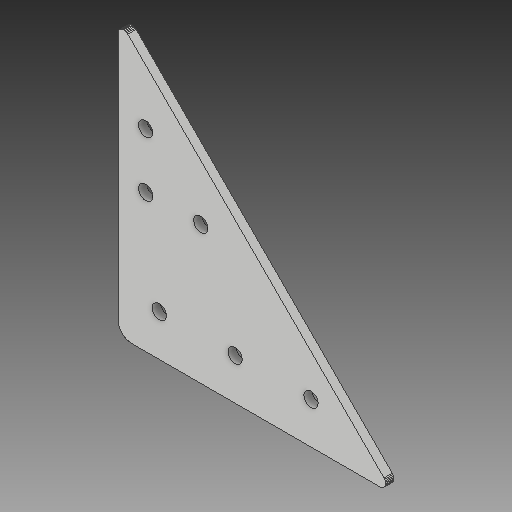
# Autodesk Inventor part: Side Brace
Saved by Autodesk Inventor 2018 (Build 220112000, 112)
## iProperties
Created: 2016-07-21
Part Number: Side Brace
Material: Generic
Document SubType Name: Modeling
Designer: User
Density: 1 g/cm^3
Appearance: Default
Author: User
Autodesk Inventor part; units mm, degrees
ref_plane "YZ Plane" through (0, 0, 0) normal (1, 0, 0) x (0, 1, 0)
ref_plane "XZ Plane" through (0, 0, 0) normal (0, 1, 0) x (-1, 0, 0)
ref_plane "XY Plane" through (0, 0, 0) normal (0, 0, 1) x (1, 0, 0)
sketch "Sketch1" plane through (0, 0, 0) normal (0, 0, 1) x (1, 0, 0)
  line L0 (141.1705, 404.7157) -> (141.0527, 405.1042)
  line L1 (141.0527, 405.1042) -> (140.8612, 405.4623)
  line L2 (140.8612, 405.4623) -> (140.6037, 405.7761)
  line L3 (140.6037, 405.7761) -> (47.6678, 498.6981)
  line L4 (47.6678, 498.6981) -> (47.354, 498.9557)
  line L5 (47.354, 498.9557) -> (46.9959, 499.1471)
  line L6 (46.9959, 499.1471) -> (46.6074, 499.265)
  line L7 (46.6074, 499.265) -> (46.2034, 499.3048)
  line L8 (46.2034, 499.3048) -> (45.7993, 499.265)
  line L9 (45.7993, 499.265) -> (45.4108, 499.1471)
  line L10 (45.4108, 499.1471) -> (45.0528, 498.9557)
  line L11 (45.0528, 498.9557) -> (44.7389, 498.6982)
  line L12 (44.7389, 498.6982) -> (44.4814, 498.3843)
  line L13 (44.4814, 498.3843) -> (44.29, 498.0263)
  line L14 (44.29, 498.0263) -> (44.1721, 497.6378)
  line L15 (44.1721, 497.6378) -> (44.1323, 497.2337)
  line L16 (44.1323, 497.2337) -> (44.1323, 407.2337)
  line L17 (44.1323, 407.2337) -> (44.1751, 406.5811)
  line L18 (44.1751, 406.5811) -> (44.3027, 405.9396)
  line L19 (44.3027, 405.9396) -> (44.5129, 405.3203)
  line L20 (44.5129, 405.3203) -> (44.8022, 404.7337)
  line L21 (44.8022, 404.7337) -> (45.1655, 404.1899)
  line L22 (45.1655, 404.1899) -> (45.5968, 403.6982)
  line L23 (45.5968, 403.6982) -> (46.0885, 403.2669)
  line L24 (46.0885, 403.2669) -> (46.6323, 402.9036)
  line L25 (46.6323, 402.9036) -> (47.2189, 402.6143)
  line L26 (47.2189, 402.6143) -> (47.8382, 402.4041)
  line L27 (47.8382, 402.4041) -> (48.4797, 402.2765)
  line L28 (48.4797, 402.2765) -> (49.1323, 402.2337)
  line L29 (49.1323, 402.2337) -> (139.1323, 402.2337)
  line L30 (139.1323, 402.2337) -> (139.5404, 402.2701)
  line L31 (139.5404, 402.2701) -> (139.929, 402.3879)
  line L32 (139.929, 402.3879) -> (140.287, 402.5794)
  line L33 (140.287, 402.5794) -> (140.6008, 402.8369)
  line L34 (140.6008, 402.8369) -> (140.8618, 403.1549)
  line L35 (140.8618, 403.1549) -> (141.0532, 403.513)
  line L36 (141.0532, 403.513) -> (141.1711, 403.9015)
  line L37 (141.1711, 403.9015) -> (141.2109, 404.3055)
  line L38 (141.2109, 404.3055) -> (141.1705, 404.7157)
  line L39 (89.0593, 417.8849) -> (88.8076, 418.4926)
  line L40 (88.8076, 418.4926) -> (88.4071, 419.0145)
  line L41 (88.4071, 419.0145) -> (87.8852, 419.415)
  line L42 (87.8852, 419.415) -> (87.2774, 419.6668)
  line L43 (87.2774, 419.6668) -> (86.6252, 419.7526)
  line L44 (86.6252, 419.7526) -> (85.973, 419.6669)
  line L45 (85.973, 419.6669) -> (85.3652, 419.4151)
  line L46 (85.3652, 419.4151) -> (84.8433, 419.0147)
  line L47 (84.8433, 419.0147) -> (84.4428, 418.4928)
  line L48 (84.4428, 418.4928) -> (84.1911, 417.885)
  line L49 (84.1911, 417.885) -> (84.1052, 417.2328)
  line L50 (84.1052, 417.2328) -> (84.191, 416.5805)
  line L51 (84.191, 416.5805) -> (84.4427, 415.9728)
  line L52 (84.4427, 415.9728) -> (84.8432, 415.4509)
  line L53 (84.8432, 415.4509) -> (85.3651, 415.0503)
  line L54 (85.3651, 415.0503) -> (85.9728, 414.7986)
  line L55 (85.9728, 414.7986) -> (86.6251, 414.7128)
  line L56 (86.6251, 414.7128) -> (87.2773, 414.7985)
  line L57 (87.2773, 414.7985) -> (87.8851, 415.0503)
  line L58 (87.8851, 415.0503) -> (88.407, 415.4507)
  line L59 (88.407, 415.4507) -> (88.8075, 415.9726)
  line L60 (88.8075, 415.9726) -> (89.0592, 416.5803)
  line L61 (89.0592, 416.5803) -> (89.1451, 417.2326)
  line L62 (89.1451, 417.2326) -> (89.0593, 417.8849)
  line L63 (61.5613, 417.885) -> (61.3095, 418.4929)
  line L64 (61.3095, 418.4929) -> (60.9091, 419.0148)
  line L65 (60.9091, 419.0148) -> (60.3872, 419.4153)
  line L66 (60.3872, 419.4153) -> (59.7794, 419.667)
  line L67 (59.7794, 419.667) -> (59.1271, 419.7529)
  line L68 (59.1271, 419.7529) -> (58.4749, 419.6671)
  line L69 (58.4749, 419.6671) -> (57.8671, 419.4154)
  line L70 (57.8671, 419.4154) -> (57.3452, 419.0149)
  line L71 (57.3452, 419.0149) -> (56.9447, 418.493)
  line L72 (56.9447, 418.493) -> (56.693, 417.8853)
  line L73 (56.693, 417.8853) -> (56.6071, 417.233)
  line L74 (56.6071, 417.233) -> (56.6929, 416.5808)
  line L75 (56.6929, 416.5808) -> (56.9446, 415.973)
  line L76 (56.9446, 415.973) -> (57.3451, 415.4511)
  line L77 (57.3451, 415.4511) -> (57.867, 415.0506)
  line L78 (57.867, 415.0506) -> (58.4748, 414.7989)
  line L79 (58.4748, 414.7989) -> (59.127, 414.713)
  line L80 (59.127, 414.713) -> (59.7792, 414.7988)
  line L81 (59.7792, 414.7988) -> (60.387, 415.0505)
  line L82 (60.387, 415.0505) -> (60.9089, 415.451)
  line L83 (60.9089, 415.451) -> (61.3094, 415.9729)
  line L84 (61.3094, 415.9729) -> (61.5611, 416.5806)
  line L85 (61.5611, 416.5806) -> (61.647, 417.233)
  line L86 (61.647, 417.233) -> (61.5613, 417.885)
  line L87 (56.5942, 452.8937) -> (56.3395, 453.5086)
  line L88 (56.3395, 453.5086) -> (55.9343, 454.0367)
  line L89 (55.9343, 454.0367) -> (55.4062, 454.4419)
  line L90 (55.4062, 454.4419) -> (54.7911, 454.6967)
  line L91 (54.7911, 454.6967) -> (54.1311, 454.7836)
  line L92 (54.1311, 454.7836) -> (53.4711, 454.6968)
  line L93 (53.4711, 454.6968) -> (52.8561, 454.4421)
  line L94 (52.8561, 454.4421) -> (52.328, 454.0368)
  line L95 (52.328, 454.0368) -> (51.9227, 453.5087)
  line L96 (51.9227, 453.5087) -> (51.668, 452.8937)
  line L97 (51.668, 452.8937) -> (51.5811, 452.2338)
  line L98 (51.5811, 452.2338) -> (51.6679, 451.5738)
  line L99 (51.6679, 451.5738) -> (51.9226, 450.9587)
  line L100 (51.9226, 450.9587) -> (52.3279, 450.4306)
  line L101 (52.3279, 450.4306) -> (52.856, 450.0253)
  line L102 (52.856, 450.0253) -> (53.471, 449.7706)
  line L103 (53.471, 449.7706) -> (54.131, 449.6837)
  line L104 (54.131, 449.6837) -> (54.791, 449.7705)
  line L105 (54.791, 449.7705) -> (55.406, 450.0252)
  line L106 (55.406, 450.0252) -> (55.9341, 450.4305)
  line L107 (55.9341, 450.4305) -> (56.3394, 450.9586)
  line L108 (56.3394, 450.9586) -> (56.5941, 451.5736)
  line L109 (56.5941, 451.5736) -> (56.681, 452.2337)
  line L110 (56.681, 452.2337) -> (56.5942, 452.8937)
  line L111 (56.597, 472.894) -> (56.3423, 473.509)
  line L112 (56.3423, 473.509) -> (55.9371, 474.0371)
  line L113 (55.9371, 474.0371) -> (55.409, 474.4424)
  line L114 (55.409, 474.4424) -> (54.794, 474.6971)
  line L115 (54.794, 474.6971) -> (54.1339, 474.784)
  line L116 (54.1339, 474.784) -> (53.4739, 474.6972)
  line L117 (53.4739, 474.6972) -> (52.8589, 474.4425)
  line L118 (52.8589, 474.4425) -> (52.3308, 474.0372)
  line L119 (52.3308, 474.0372) -> (51.9255, 473.5091)
  line L120 (51.9255, 473.5091) -> (51.6708, 472.8941)
  line L121 (51.6708, 472.8941) -> (51.5839, 472.2341)
  line L122 (51.5839, 472.2341) -> (51.6707, 471.5741)
  line L123 (51.6707, 471.5741) -> (51.9254, 470.9591)
  line L124 (51.9254, 470.9591) -> (52.3307, 470.431)
  line L125 (52.3307, 470.431) -> (52.8588, 470.0257)
  line L126 (52.8588, 470.0257) -> (53.4738, 469.771)
  line L127 (53.4738, 469.771) -> (54.1337, 469.6841)
  line L128 (54.1337, 469.6841) -> (54.7938, 469.7709)
  line L129 (54.7938, 469.7709) -> (55.4087, 470.0256)
  line L130 (55.4087, 470.0256) -> (55.9369, 470.4309)
  line L131 (55.9369, 470.4309) -> (56.3422, 470.959)
  line L132 (56.3422, 470.959) -> (56.5969, 471.574)
  line L133 (56.5969, 471.574) -> (56.6838, 472.2341)
  line L134 (56.6838, 472.2341) -> (56.597, 472.894)
  line L135 (76.5952, 452.8937) -> (76.3405, 453.5086)
  line L136 (76.3405, 453.5086) -> (75.9352, 454.0368)
  line L137 (75.9352, 454.0368) -> (75.4071, 454.442)
  line L138 (75.4071, 454.442) -> (74.7921, 454.6968)
  line L139 (74.7921, 454.6968) -> (74.1322, 454.7837)
  line L140 (74.1322, 454.7837) -> (73.4722, 454.6969)
  line L141 (73.4722, 454.6969) -> (72.8571, 454.4421)
  line L142 (72.8571, 454.4421) -> (72.329, 454.0369)
  line L143 (72.329, 454.0369) -> (71.9237, 453.5088)
  line L144 (71.9237, 453.5088) -> (71.669, 452.8938)
  line L145 (71.669, 452.8938) -> (71.5821, 452.2338)
  line L146 (71.5821, 452.2338) -> (71.6689, 451.5738)
  line L147 (71.6689, 451.5738) -> (71.9237, 450.9588)
  line L148 (71.9237, 450.9588) -> (72.3289, 450.4307)
  line L149 (72.3289, 450.4307) -> (72.857, 450.0254)
  line L150 (72.857, 450.0254) -> (73.472, 449.7706)
  line L151 (73.472, 449.7706) -> (74.132, 449.6838)
  line L152 (74.132, 449.6838) -> (74.792, 449.7705)
  line L153 (74.792, 449.7705) -> (75.407, 450.0253)
  line L154 (75.407, 450.0253) -> (75.9352, 450.4305)
  line L155 (75.9352, 450.4305) -> (76.3404, 450.9586)
  line L156 (76.3404, 450.9586) -> (76.5952, 451.5736)
  line L157 (76.5952, 451.5736) -> (76.682, 452.2334)
  line L158 (76.682, 452.2334) -> (76.5952, 452.8937)
  line L159 (116.5587, 417.8849) -> (116.307, 418.4926)
  line L160 (116.307, 418.4926) -> (115.9066, 419.0145)
  line L161 (115.9066, 419.0145) -> (115.3847, 419.415)
  line L162 (115.3847, 419.415) -> (114.7769, 419.6667)
  line L163 (114.7769, 419.6667) -> (114.1247, 419.7526)
  line L164 (114.1247, 419.7526) -> (113.4724, 419.6668)
  line L165 (113.4724, 419.6668) -> (112.8647, 419.415)
  line L166 (112.8647, 419.415) -> (112.3428, 419.0146)
  line L167 (112.3428, 419.0146) -> (111.9423, 418.4927)
  line L168 (111.9423, 418.4927) -> (111.6905, 417.8849)
  line L169 (111.6905, 417.8849) -> (111.6047, 417.2327)
  line L170 (111.6047, 417.2327) -> (111.6904, 416.5804)
  line L171 (111.6904, 416.5804) -> (111.9422, 415.9727)
  line L172 (111.9422, 415.9727) -> (112.3426, 415.4508)
  line L173 (112.3426, 415.4508) -> (112.8645, 415.0503)
  line L174 (112.8645, 415.0503) -> (113.4723, 414.7986)
  line L175 (113.4723, 414.7986) -> (114.1246, 414.7127)
  line L176 (114.1246, 414.7127) -> (114.7768, 414.7985)
  line L177 (114.7768, 414.7985) -> (115.3846, 415.0502)
  line L178 (115.3846, 415.0502) -> (115.9065, 415.4507)
  line L179 (115.9065, 415.4507) -> (116.307, 415.9726)
  line L180 (116.307, 415.9726) -> (116.5587, 416.5802)
  line L181 (116.5587, 416.5802) -> (116.6445, 417.2325)
  line L182 (116.6445, 417.2325) -> (116.5587, 417.8849)
  point P0 (0, 0)
  constraints: 366 end point, 13 perpendicular, 2 parallel
extrude "Extrusion1" add sketch "Sketch1" along normal blind 3
sketch "Sketch2" plane through (0, 0, 0) normal (0, 0, -1) x (-1, 0, 0)
  line L0 (-56.6838, 472.2341) -> (-56.597, 472.894) projected
  line L1 (-56.597, 472.894) -> (-56.3423, 473.509) projected
  line L2 (-56.3423, 473.509) -> (-55.9371, 474.0371) projected
  line L3 (-55.9371, 474.0371) -> (-55.409, 474.4424) projected
  line L4 (-55.409, 474.4424) -> (-54.794, 474.6971) projected
  line L5 (-54.794, 474.6971) -> (-54.1339, 474.784) projected
  line L6 (-54.1339, 474.784) -> (-53.4739, 474.6972) projected
  line L7 (-53.4739, 474.6972) -> (-52.8589, 474.4425) projected
  line L8 (-52.8589, 474.4425) -> (-52.3308, 474.0372) projected
  line L9 (-52.3308, 474.0372) -> (-51.9255, 473.5091) projected
  line L10 (-51.9255, 473.5091) -> (-51.6708, 472.8941) projected
  line L11 (-51.6708, 472.8941) -> (-51.5839, 472.2341) projected
  line L12 (-51.5839, 472.2341) -> (-51.6707, 471.5741) projected
  line L13 (-51.6707, 471.5741) -> (-51.9254, 470.9591) projected
  line L14 (-51.9254, 470.9591) -> (-52.3307, 470.431) projected
  line L15 (-52.3307, 470.431) -> (-52.8588, 470.0257) projected
  line L16 (-52.8588, 470.0257) -> (-53.4738, 469.771) projected
  line L17 (-53.4738, 469.771) -> (-54.1337, 469.6841) projected
  line L18 (-54.1337, 469.6841) -> (-54.7938, 469.7709) projected
  line L19 (-54.7938, 469.7709) -> (-55.4087, 470.0256) projected
  line L20 (-55.4087, 470.0256) -> (-55.9369, 470.4309) projected
  line L21 (-55.9369, 470.4309) -> (-56.3422, 470.959) projected
  line L22 (-56.3422, 470.959) -> (-56.5969, 471.574) projected
  line L23 (-56.5969, 471.574) -> (-56.6838, 472.2341) projected
  line L24 (-76.682, 452.2334) -> (-76.5952, 452.8937) projected
  line L25 (-76.5952, 452.8937) -> (-76.3405, 453.5086) projected
  line L26 (-76.3405, 453.5086) -> (-75.9352, 454.0368) projected
  line L27 (-75.9352, 454.0368) -> (-75.4071, 454.442) projected
  line L28 (-75.4071, 454.442) -> (-74.7921, 454.6968) projected
  line L29 (-74.7921, 454.6968) -> (-74.1322, 454.7837) projected
  line L30 (-74.1322, 454.7837) -> (-73.4722, 454.6969) projected
  line L31 (-73.4722, 454.6969) -> (-72.8571, 454.4421) projected
  line L32 (-72.8571, 454.4421) -> (-72.329, 454.0369) projected
  line L33 (-72.329, 454.0369) -> (-71.9237, 453.5088) projected
  line L34 (-71.9237, 453.5088) -> (-71.669, 452.8938) projected
  line L35 (-71.669, 452.8938) -> (-71.5821, 452.2338) projected
  line L36 (-71.5821, 452.2338) -> (-71.6689, 451.5738) projected
  line L37 (-71.6689, 451.5738) -> (-71.9237, 450.9588) projected
  line L38 (-71.9237, 450.9588) -> (-72.3289, 450.4307) projected
  line L39 (-72.3289, 450.4307) -> (-72.857, 450.0254) projected
  line L40 (-72.857, 450.0254) -> (-73.472, 449.7706) projected
  line L41 (-73.472, 449.7706) -> (-74.132, 449.6838) projected
  line L42 (-74.132, 449.6838) -> (-74.792, 449.7705) projected
  line L43 (-74.792, 449.7705) -> (-75.407, 450.0253) projected
  line L44 (-75.407, 450.0253) -> (-75.9352, 450.4305) projected
  line L45 (-75.9352, 450.4305) -> (-76.3404, 450.9586) projected
  line L46 (-76.3404, 450.9586) -> (-76.5952, 451.5736) projected
  line L47 (-76.5952, 451.5736) -> (-76.682, 452.2334) projected
  line L48 (-56.681, 452.2337) -> (-56.5942, 452.8937) projected
  line L49 (-56.5942, 452.8937) -> (-56.3395, 453.5086) projected
  line L50 (-56.3395, 453.5086) -> (-55.9343, 454.0367) projected
  line L51 (-55.9343, 454.0367) -> (-55.4062, 454.4419) projected
  line L52 (-55.4062, 454.4419) -> (-54.7911, 454.6967) projected
  line L53 (-54.7911, 454.6967) -> (-54.1311, 454.7836) projected
  line L54 (-54.1311, 454.7836) -> (-53.4711, 454.6968) projected
  line L55 (-53.4711, 454.6968) -> (-52.8561, 454.4421) projected
  line L56 (-52.8561, 454.4421) -> (-52.328, 454.0368) projected
  line L57 (-52.328, 454.0368) -> (-51.9227, 453.5087) projected
  line L58 (-51.9227, 453.5087) -> (-51.668, 452.8937) projected
  line L59 (-51.668, 452.8937) -> (-51.5811, 452.2338) projected
  line L60 (-51.5811, 452.2338) -> (-51.6679, 451.5738) projected
  line L61 (-51.6679, 451.5738) -> (-51.9226, 450.9587) projected
  line L62 (-51.9226, 450.9587) -> (-52.3279, 450.4306) projected
  line L63 (-52.3279, 450.4306) -> (-52.856, 450.0253) projected
  line L64 (-52.856, 450.0253) -> (-53.471, 449.7706) projected
  line L65 (-53.471, 449.7706) -> (-54.131, 449.6837) projected
  line L66 (-54.131, 449.6837) -> (-54.791, 449.7705) projected
  line L67 (-54.791, 449.7705) -> (-55.406, 450.0252) projected
  line L68 (-55.406, 450.0252) -> (-55.9341, 450.4305) projected
  line L69 (-55.9341, 450.4305) -> (-56.3394, 450.9586) projected
  line L70 (-56.3394, 450.9586) -> (-56.5941, 451.5736) projected
  line L71 (-56.5941, 451.5736) -> (-56.681, 452.2337) projected
  line L72 (-89.1451, 417.2326) -> (-89.0593, 417.8849) projected
  line L73 (-89.0593, 417.8849) -> (-88.8076, 418.4926) projected
  line L74 (-88.8076, 418.4926) -> (-88.4071, 419.0145) projected
  line L75 (-88.4071, 419.0145) -> (-87.8852, 419.415) projected
  line L76 (-87.8852, 419.415) -> (-87.2774, 419.6668) projected
  line L77 (-87.2774, 419.6668) -> (-86.6252, 419.7526) projected
  line L78 (-86.6252, 419.7526) -> (-85.973, 419.6669) projected
  line L79 (-85.973, 419.6669) -> (-85.3652, 419.4151) projected
  line L80 (-85.3652, 419.4151) -> (-84.8433, 419.0147) projected
  line L81 (-84.8433, 419.0147) -> (-84.4428, 418.4928) projected
  line L82 (-84.4428, 418.4928) -> (-84.1911, 417.885) projected
  line L83 (-84.1911, 417.885) -> (-84.1052, 417.2328) projected
  line L84 (-84.1052, 417.2328) -> (-84.191, 416.5805) projected
  line L85 (-84.191, 416.5805) -> (-84.4427, 415.9728) projected
  line L86 (-84.4427, 415.9728) -> (-84.8432, 415.4509) projected
  line L87 (-84.8432, 415.4509) -> (-85.3651, 415.0503) projected
  line L88 (-85.3651, 415.0503) -> (-85.9728, 414.7986) projected
  line L89 (-85.9728, 414.7986) -> (-86.6251, 414.7128) projected
  line L90 (-86.6251, 414.7128) -> (-87.2773, 414.7985) projected
  line L91 (-87.2773, 414.7985) -> (-87.8851, 415.0503) projected
  line L92 (-87.8851, 415.0503) -> (-88.407, 415.4507) projected
  line L93 (-88.407, 415.4507) -> (-88.8075, 415.9726) projected
  line L94 (-88.8075, 415.9726) -> (-89.0592, 416.5803) projected
  line L95 (-89.0592, 416.5803) -> (-89.1451, 417.2326) projected
  line L96 (-61.647, 417.233) -> (-61.5613, 417.885) projected
  line L97 (-61.5613, 417.885) -> (-61.3095, 418.4929) projected
  line L98 (-61.3095, 418.4929) -> (-60.9091, 419.0148) projected
  line L99 (-60.9091, 419.0148) -> (-60.3872, 419.4153) projected
  line L100 (-60.3872, 419.4153) -> (-59.7794, 419.667) projected
  line L101 (-59.7794, 419.667) -> (-59.1271, 419.7529) projected
  line L102 (-59.1271, 419.7529) -> (-58.4749, 419.6671) projected
  line L103 (-58.4749, 419.6671) -> (-57.8671, 419.4154) projected
  line L104 (-57.8671, 419.4154) -> (-57.3452, 419.0149) projected
  line L105 (-57.3452, 419.0149) -> (-56.9447, 418.493) projected
  line L106 (-56.9447, 418.493) -> (-56.693, 417.8853) projected
  line L107 (-56.693, 417.8853) -> (-56.6071, 417.233) projected
  line L108 (-56.6071, 417.233) -> (-56.6929, 416.5808) projected
  line L109 (-56.6929, 416.5808) -> (-56.9446, 415.973) projected
  line L110 (-56.9446, 415.973) -> (-57.3451, 415.4511) projected
  line L111 (-57.3451, 415.4511) -> (-57.867, 415.0506) projected
  line L112 (-57.867, 415.0506) -> (-58.4748, 414.7989) projected
  line L113 (-58.4748, 414.7989) -> (-59.127, 414.713) projected
  line L114 (-59.127, 414.713) -> (-59.7792, 414.7988) projected
  line L115 (-59.7792, 414.7988) -> (-60.387, 415.0505) projected
  line L116 (-60.387, 415.0505) -> (-60.9089, 415.451) projected
  line L117 (-60.9089, 415.451) -> (-61.3094, 415.9729) projected
  line L118 (-61.3094, 415.9729) -> (-61.5611, 416.5806) projected
  line L119 (-61.5611, 416.5806) -> (-61.647, 417.233) projected
  line L120 (-116.6445, 417.2325) -> (-116.5587, 417.8849) projected
  line L121 (-116.5587, 417.8849) -> (-116.307, 418.4926) projected
  line L122 (-116.307, 418.4926) -> (-115.9066, 419.0145) projected
  line L123 (-115.9066, 419.0145) -> (-115.3847, 419.415) projected
  line L124 (-115.3847, 419.415) -> (-114.7769, 419.6667) projected
  line L125 (-114.7769, 419.6667) -> (-114.1247, 419.7526) projected
  line L126 (-114.1247, 419.7526) -> (-113.4724, 419.6668) projected
  line L127 (-113.4724, 419.6668) -> (-112.8647, 419.415) projected
  line L128 (-112.8647, 419.415) -> (-112.3428, 419.0146) projected
  line L129 (-112.3428, 419.0146) -> (-111.9423, 418.4927) projected
  line L130 (-111.9423, 418.4927) -> (-111.6905, 417.8849) projected
  line L131 (-111.6905, 417.8849) -> (-111.6047, 417.2327) projected
  line L132 (-111.6047, 417.2327) -> (-111.6904, 416.5804) projected
  line L133 (-111.6904, 416.5804) -> (-111.9422, 415.9727) projected
  line L134 (-111.9422, 415.9727) -> (-112.3426, 415.4508) projected
  line L135 (-112.3426, 415.4508) -> (-112.8645, 415.0503) projected
  line L136 (-112.8645, 415.0503) -> (-113.4723, 414.7986) projected
  line L137 (-113.4723, 414.7986) -> (-114.1246, 414.7127) projected
  line L138 (-114.1246, 414.7127) -> (-114.7768, 414.7985) projected
  line L139 (-114.7768, 414.7985) -> (-115.3846, 415.0502) projected
  line L140 (-115.3846, 415.0502) -> (-115.9065, 415.4507) projected
  line L141 (-115.9065, 415.4507) -> (-116.307, 415.9726) projected
  line L142 (-116.307, 415.9726) -> (-116.5587, 416.5802) projected
  line L143 (-116.5587, 416.5802) -> (-116.6445, 417.2325) projected
  line L144 (-141.1705, 404.7157) -> (-141.0527, 405.1042) projected
  line L145 (-141.2109, 404.3055) -> (-141.1705, 404.7157) projected
  line L146 (-141.1711, 403.9015) -> (-141.2109, 404.3055) projected
  line L147 (-141.0532, 403.513) -> (-141.1711, 403.9015) projected
  line L148 (-140.8618, 403.1549) -> (-141.0532, 403.513) projected
  line L149 (-140.6008, 402.8369) -> (-140.8618, 403.1549) projected
  line L150 (-140.287, 402.5794) -> (-140.6008, 402.8369) projected
  line L151 (-139.929, 402.3879) -> (-140.287, 402.5794) projected
  line L152 (-139.5404, 402.2701) -> (-139.929, 402.3879) projected
  line L153 (-139.1323, 402.2337) -> (-139.5404, 402.2701) projected
  line L154 (-49.1323, 402.2337) -> (-139.1323, 402.2337) projected
  line L155 (-48.4797, 402.2765) -> (-49.1323, 402.2337) projected
  line L156 (-47.8382, 402.4041) -> (-48.4797, 402.2765) projected
  line L157 (-47.2189, 402.6143) -> (-47.8382, 402.4041) projected
  line L158 (-46.6323, 402.9036) -> (-47.2189, 402.6143) projected
  line L159 (-46.0885, 403.2669) -> (-46.6323, 402.9036) projected
  line L160 (-45.5968, 403.6982) -> (-46.0885, 403.2669) projected
  line L161 (-45.1655, 404.1899) -> (-45.5968, 403.6982) projected
  line L162 (-44.8022, 404.7337) -> (-45.1655, 404.1899) projected
  line L163 (-44.5129, 405.3203) -> (-44.8022, 404.7337) projected
  line L164 (-44.3027, 405.9396) -> (-44.5129, 405.3203) projected
  line L165 (-44.1751, 406.5811) -> (-44.3027, 405.9396) projected
  line L166 (-44.1323, 407.2337) -> (-44.1751, 406.5811) projected
  line L167 (-44.1323, 497.2337) -> (-44.1323, 407.2337) projected
  line L168 (-44.1721, 497.6378) -> (-44.1323, 497.2337) projected
  line L169 (-44.29, 498.0263) -> (-44.1721, 497.6378) projected
  line L170 (-44.4814, 498.3843) -> (-44.29, 498.0263) projected
  line L171 (-44.7389, 498.6982) -> (-44.4814, 498.3843) projected
  line L172 (-45.0528, 498.9557) -> (-44.7389, 498.6982) projected
  line L173 (-45.4108, 499.1471) -> (-45.0528, 498.9557) projected
  line L174 (-45.7993, 499.265) -> (-45.4108, 499.1471) projected
  line L175 (-46.2034, 499.3048) -> (-45.7993, 499.265) projected
  line L176 (-46.6074, 499.265) -> (-46.2034, 499.3048) projected
  line L177 (-46.9959, 499.1471) -> (-46.6074, 499.265) projected
  line L178 (-47.354, 498.9557) -> (-46.9959, 499.1471) projected
  line L179 (-47.6678, 498.6981) -> (-47.354, 498.9557) projected
  line L180 (-140.6037, 405.7761) -> (-47.6678, 498.6981) projected
  line L181 (-140.8612, 405.4623) -> (-140.6037, 405.7761) projected
  line L182 (-141.0527, 405.1042) -> (-140.8612, 405.4623) projected
  circle A0 centre (-54.1338, 472.234) radius 2.5282
  circle A1 centre (-54.1311, 452.2337) radius 2.5282
  circle A2 centre (-74.1321, 452.2337) radius 2.5282
  circle A3 centre (-86.6252, 417.2327) radius 2.4985
  circle A4 centre (-114.1247, 417.2326) radius 2.4984
  circle A5 centre (-59.1271, 417.2329) radius 2.4984
  point P0 (0, 0)
  constraints: 18 tangent, 6 centre point
hole "Hole1" at (114.1247, 417.2326, 0) at (86.6252, 417.2327, 0) at (59.1271, 417.2329, 0) at (54.1311, 452.2337, 0) at (74.1321, 452.2337, 0) at (54.1338, 472.234, 0) direction (0, 0, 1) diameter 5.2 end through all
body "Solid1"
